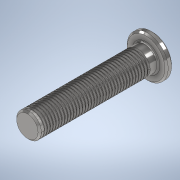
# Autodesk Inventor part: Parafuso1.5_2
Saved by Autodesk Inventor 2021 (Build 250183000, 183)
## iProperties
Created: 2020-12-04
Part Number: Parafuso1.5_2
Material: Steel
Document SubType Name: Modeling
Designer: Lucas Moura
Density: 7.85 g/cm^3
Appearance: Steel - Polished
Author: Lucas Moura
Autodesk Inventor part; units mm, degrees
ref_plane "YZ Plane" through (0, 0, 0) normal (1, 0, 0) x (0, 1, 0)
ref_plane "XZ Plane" through (0, 0, 0) normal (0, 1, 0) x (-1, 0, 0)
ref_plane "XY Plane" through (0, 0, 0) normal (0, 0, 1) x (1, 0, 0)
sketch "Sketch3" plane through (0, 0, 0) normal (0, 0, 1) x (1, 0, 0)
  circle A0 centre (0, 0) radius 0.75
  dimension "d6" = 1.5
  constraints: 1 centre point, 1 coincident
  measures "d6" diameter of A0
extrude "Extrusion3" add sketch "Sketch3" along normal blind 7.23
chamfer "Chamfer1" distance 0.1 angle 45 1 edges at (-0.75, 0, 7.23)
sketch "Sketch4" plane through (0, 0, 0) normal (0, 0, -1) x (-1, 0, 0)
  circle A0 centre (0, 0) radius 1.25
  dimension "d12" = 2.5
  constraints: 1 centre point, 1 coincident
  measures "d12" diameter of A0
extrude "Extrusion4" add sketch "Sketch4" along normal blind 0.4
fillet "Fillet1" radius 0.1 1 edges at (-0.75, 0, 0)
chamfer "Chamfer2" distance 0.1 angle 45 1 edges at (1.25, 0, -0.4)
chamfer "Chamfer3" distance 0.1 angle 45 1 edges at (1.25, 0, 0)
sketch "Sketch5" plane through (0, 0, -0.4) normal (0, 0, -1) x (-1, 0, 0)
  line L0 (0.7348, -0.15) -> (-0.7348, -0.15)
  line L1 (-0.7348, -0.15) -> (-0.7348, 0.15)
  line L2 (-0.7348, 0.15) -> (0.7348, 0.15)
  line L3 (0.7348, 0.15) -> (0.7348, -0.15)
  line L4 (0.7348, -0.15) -> (-0.7348, 0.15) construction
  line L5 (-0.7348, -0.15) -> (0.7348, 0.15) construction
  line L6 (0.15, -0.75) -> (-0.15, -0.75)
  line L7 (-0.15, -0.75) -> (-0.15, 0.75)
  line L8 (-0.15, 0.75) -> (0.15, 0.75)
  line L9 (0.15, 0.75) -> (0.15, -0.75)
  line L10 (0.15, -0.75) -> (-0.15, 0.75) construction
  line L11 (-0.15, -0.75) -> (0.15, 0.75) construction
  point P0 (0, 0)
  point P1 (-0.15, -0.15)
  point P2 (0.15, -0.15)
  point P3 (0.15, 0.15)
  point P4 (-0.15, 0.15)
  dimension "d25" = 0.3
  dimension "d26" = 0.3
  dimension "d27" = 1.5
  constraints: 24 end point, 4 midpoint, 4 parallel, 2 horizontal, 2 perpendicular
  measures "d25" distance of L0.end L1.end
  measures "d26" distance of L7.end L8.end
  measures "d27" distance of L6.end L7.end
extrude "Extrusion5" cut sketch "Sketch5" against normal blind 0.2
sketch "Sketch6" plane through (0, 0, 0) normal (0, 1, 0) x (-1, 0, 0)
  line L0 (0, -1.547) -> (0, 9.282) projected
  line L1 (-0.75, 0.1) -> (-0.75, 7.13) construction
  line L2 (0.85, 0) -> (-0.85, 0) projected
  line L3 (-0.75, 0.5) -> (-0.5255, 0.5) construction
  line L4 (-0.75, 0.5) -> (-0.6634, 0.55)
  line L5 (-0.6634, 0.55) -> (-0.6634, 0.6) construction
  line L6 (-0.6634, 0.6) -> (-0.75, 0.65)
  line L7 (-0.75, 0.5) -> (-0.75, 0.65) construction
  line L8 (-0.7067, 0.525) -> (-0.7067, 0.625) construction
  arc A0 (-0.6634, 0.55) -> (-0.6634, 0.6) centre (-0.6778, 0.575) ccw
  line L9 (-0.75, 0.5) -> (-0.75, 0.65)
  point P0 (0, 0)
  dimension "d32" = 0.5
  dimension "d33" = 60
  dimension "d35" = 0.1
  dimension "d36" = 0.05
  constraints: 14 end point, 2 midpoint, 2 point on circle, 2 point on line, 2 tangent, 1 centre point, 1 collinear, 1 equal length, 1 parallel, 1 vertical
  measures "d32" distance between parallel lines of L2 L3
  measures "d33" angle of L6 L4
  measures "d35" distance of L8.start L8.end
  measures "d36" distance of L4.end L5.end
coil "Coil1" sketch "Sketch6" operation cut axis through (0, 0, -10) along (0, 0, 1) pitch 0.18 turns 36 hand right
fillet "Fillet3" radius 0.1 4 edges at (0.15, -0.15, -0.3) (-0.15, -0.15, -0.3) (-0.15, 0.15, -0.3) (0.15, 0.15, -0.3)
sketch "Sketch7" plane through (0.6778, 0, 0.575) normal (0, 1, 0) x (1, 0, 0)
  line L0 (0.0722, 0.075) -> (-0.0144, 0.025) projected
  arc A0 (-0.0144, 0.025) -> (-0.0144, -0.025) centre (0, 0) ccw projected
  line L1 (-0.0144, -0.025) -> (0.0722, -0.075) projected
  line L2 (0.0722, 0.075) -> (0.0722, -0.075) projected
  point P0 (-0.6778, 0.575)
extrude "Extrusion6" cut sketch "Sketch7" against normal blind 0.6
equation "\"d36\" = 0.5 * d35"
body "Solid2"
